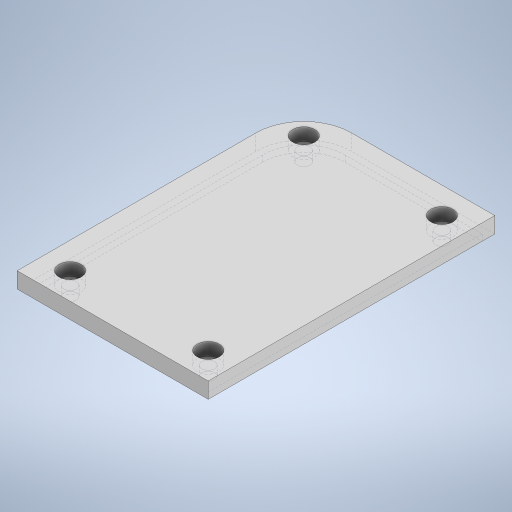
# Autodesk Inventor part: Deckel_Gehäuse
Saved by Autodesk Inventor 2024.2 (Build 282272000, 272)
## iProperties
Created: 2023-10-24
Part Number: Deckel_Gehäuse
Material: Generisch
Document SubType Name: Modeling
Designer: Pieber
Density: 1 g/cm^3
Appearance: Vorgabe
Author: Pieber
Autodesk Inventor part; units mm, degrees
ref_plane "YZ Plane" through (0, 0, 0) normal (1, 0, 0) x (0, 1, 0)
ref_plane "XZ Plane" through (0, 0, 0) normal (0, 1, 0) x (-1, 0, 0)
ref_plane "XY Plane" through (0, 0, 0) normal (0, 0, 1) x (1, 0, 0)
sketch "Skizze16" plane through (0, 0, 0) normal (0, 0, 1) x (1, 0, 0)
  line L0 (-30, 45) -> (30, 45)
  line L1 (30, 45) -> (30, -45)
  line L2 (30, -45) -> (-30, -45)
  line L3 (-30, -45) -> (-30, 45)
  line L4 (-30, 45) -> (30, -45) construction
  line L5 (30, 45) -> (-30, -45) construction
  point P0 (0, 0)
  dimension "d50" = 60
  dimension "d51" = 90
  constraints: 12 end point, 2 midpoint, 2 parallel, 1 horizontal, 1 perpendicular
  measures "d50" distance of L1.end L2.end
  measures "d51" distance of L0.end L1.end
extrude "Extrusion13" add sketch "Skizze16" along normal blind 5
fillet "Rundung1" radius 15 1 edges at (-30, 45, 2.5)
sketch "Skizze22" plane through (0, 0, 0) normal (0, 0, -1) x (-1, 0, 0)
  line L0 (30, -45) -> (-30, -45) projected
  line L1 (30, -45) -> (28, -45)
  line L2 (28, -45) -> (28, 30)
  line L3 (28, 30) -> (30, 30)
  line L4 (30, 30) -> (30, -45)
  line L5 (-30, -45) -> (28, -45)
  line L6 (28, -45) -> (28, -43)
  line L7 (28, -43) -> (-30, -43)
  line L8 (-30, -43) -> (-30, -45)
  line L9 (-30, 45) -> (15, 45) projected
  line L10 (-30, -43) -> (-28, -43)
  line L11 (-28, -43) -> (-28, 45)
  line L12 (-28, 45) -> (-30, 45)
  line L13 (-30, 45) -> (-30, -43)
  line L14 (-28, 45) -> (15, 45)
  line L15 (15, 45) -> (15, 43)
  line L16 (15, 43) -> (-28, 43)
  line L17 (-28, 43) -> (-28, 45)
  arc A0 (30, 30) -> (15, 45) centre (15, 30) ccw
  arc A1 (28, 30) -> (15, 43) centre (15, 30) ccw
  point P0 (0, 0)
  dimension "d92" = 2
  dimension "d93" = 75
  dimension "d94" = 2
  dimension "d95" = 2
  dimension "d96" = 2
  constraints: 32 end point, 8 parallel, 4 horizontal, 4 perpendicular, 4 point on circle, 2 centre point, 2 point on line, 1 coincident
  measures "d92" distance of L2.end L3.end
  measures "d93" distance of L1.end L2.end
  measures "d94" distance of L6.end L5.end
  measures "d95" distance of L12.end L11.end
  measures "d96" distance of L14.end L15.end
extrude "Extrusion17" add sketch "Skizze22" along normal blind 2 contours L7 L11 L16 A1 L2
sketch "Skizze23" plane through (0, 0, 5) normal (0, 0, 1) x (1, 0, 0)
  circle A0 centre (21.7, -36.7) radius 2
  line L0 (30, -45) -> (30, 45) projected
  line L1 (-30, -45) -> (30, -45) projected
  point P0 (0, 0)
  dimension "d99" = 4
  dimension "d100" = 8.3
  dimension "d101" = 8.3
  constraints: 1 centre point
  measures "d99" diameter of A0
  measures "d100" distance from line of A0.centre L0
  measures "d101" distance from line of A0.centre L1
extrude "Extrusion18" cut sketch "Skizze23" against normal through all
sketch "Skizze24" plane through (0, 0, 5) normal (0, 0, 1) x (1, 0, 0)
  circle A0 centre (21.7, -36.7) radius 2 projected
  circle A1 centre (21.7, -36.7) radius 3.5
  point P0 (0, 0)
  dimension "d104" = 7
  constraints: 1 centre point, 1 coincident
  measures "d104" diameter of A1
extrude "Extrusion19" cut sketch "Skizze24" against normal blind 4
mirror "Spiegeln5" about plane through (0, 0, 0) normal (0, 1, 0) of "Extrusion19", "Extrusion18"
mirror "Spiegeln6" about plane through (0, 0, 0) normal (1, 0, 0) of "Extrusion19", "Extrusion18", "Spiegeln5"
